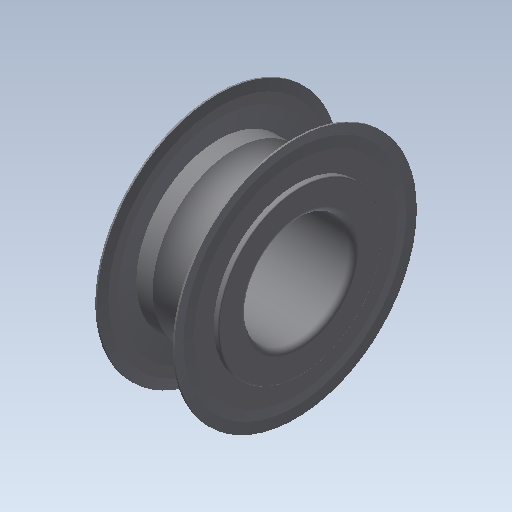
# Autodesk Inventor part: 6201-2Z_PART1
Saved by Autodesk Inventor 2020 (Build 240168000, 168)
## iProperties
Created: 2019-03-20
Part Number: 6201-2Z_PART1
Material: Generic
Catalog Web Link: www.cadenas.de
Description: -Deep groove ball bearings
Vendor: SKF
Document SubType Name: Modeling
Designer: psadmin
Manufacturer: SKF
Mass: 1.48168 g
Surface Area: 25.5062 cm^2
Volume: 1.48168 cm^3
Density: 1 g/cm^3
Appearance: PSOLRGB-175-175-175
Category: PARTsolutions
Company: SKF
PSOL_IDENT_0: {$CADENAS_DATA\23d-libs\skf\bearings_units_and_housings\ball_bearings\deep_groove_ball_bearings\bb1_
PSOL_IDENT_1: 001_101.prj},192 {VTYP=3D},{NB=6201-2Z_PART1},{LINA=6201-2Z_PART1},{NN=BB1_001_101_PART1},{NOPRJ=TRU
PSOL_IDENT_2: E},{DATE=18.03.2019 09:24:30},{GEOMDATE=08.08.2018 12:16:40},{VERSION=},{LINEID=9770},{WBVAR=},{WBNU
PSOL_IDENT_3: MERIC=}  {NB=6201-2Z_PART1},{LINA=6201-2Z_PART1},{KT=DUMMY},{PRODUCTID=1050070201},{DESIGNATION=6201
PSOL_IDENT_4: -2Z},{DD=12.00},{D=32.000},{B=10.000},{C=0.000},{DD1=18.45},{DD2=0.0},{D1=0.00},{D2=27.34},{D3=0.00}
PSOL_IDENT_5: ,{D4=0.000},{HH=MIN},{BB=0.000},{FF=0.00},{R0MAX=MIN},{R0=MIN},{R12=0.60},{PITCH=22.00},{DW=6.000},{
PSOL_IDENT_6: DDAMIN=16.200},{DDAMAX=18.400},{DDBMIN=MIN},{DDBMAX=MIN},{DBMIN=MIN},{DAMAX=27.800},{BBAMIN=MIN},{CA
PSOL_IDENT_7: MAX=MIN},{RAMAX=0.600},{LOAD1=7.280},{LOAD2=3.100},{LOAD3=0.132},{SPEED1=50000},{SPEED2=26000},{KR=0
PSOL_IDENT_8: .025},{F0=12.000},{Z=7},{II=1},{MASS=0.039},{BEARING=6201-2Z},{RING=},{HELP=2.990},{HELP2=2.330},{DD
PSOL_IDENT_9: 1ALG=9.225},{YALG=9.225},{PITCH1=22.000},{DW1=6.000},{YALG1=13.010},{HALG1=2.990},{SH=9.225},{CU=0.8
PSOL_IDENT_10: 00},{DESIGN=dgbbw2z},{HALG=3.225},{B1=0},{ALGO=1.000}
NT: Deep groove ball bearings
NB: 6201-2Z_PART1
NBSYN: $DESIGNATION._PART1
LINA: 6201-2Z_PART1
SUPPLIER: SKF
ARTICLENO: 6201-2Z_PART1
BOMINFO: 6201-2Z_PART1
CREATOR: CADENAS GmbH
Title: 6201-2Z_PART1
Author: Cadenas PARTsolutions
Comments: Deep groove ball bearings
Autodesk Inventor part; units mm, degrees
ref_plane "YZ Plane" through (0, 0, 0) normal (1, 0, 0) x (0, 1, 0)
ref_plane "XZ Plane" through (0, 0, 0) normal (0, 1, 0) x (-1, 0, 0)
ref_plane "XY Plane" through (0, 0, 0) normal (0, 0, 1) x (1, 0, 0)
sketch "Sketch_17" plane through (0, 0, 0) normal (0, 0, 1) x (1, 0, 0)
  line L0 (50, 0) -> (-50, 0)
  line L1 (0, 9.105) -> (0, 6.6)
  arc A0 (0, 6.6) -> (0.6, 6) centre (0.6, 6.6) ccw
  line L2 (0.6, 6) -> (9.4, 6)
  arc A1 (9.4, 6) -> (10, 6.6) centre (9.4, 6.6) ccw
  line L3 (10, 6.6) -> (10, 9.105)
  arc A2 (10, 9.105) -> (9.88, 9.225) centre (9.88, 9.105) ccw
  line L4 (9.88, 9.225) -> (7.4185, 9.225)
  arc A3 (2.5815, 9.225) -> (7.4185, 9.225) centre (5, 11) ccw
  line L5 (2.5815, 9.225) -> (0.12, 9.225)
  arc A4 (0.12, 9.225) -> (0, 9.105) centre (0.12, 9.105) ccw
  constraints: 12 end point, 10 point on circle, 5 centre point
revolve "Revolution1" add sketch "Sketch_17" angle 360 about axis through (50, 0, 0) along (1, 0, 0)
sketch "Sketch_20" plane through (0, 0, 0) normal (0, 0, 1) x (1, 0, 0)
  line L0 (50, 0) -> (-50, 0)
  line L1 (0.54, 13.67) -> (0.63, 12.5563)
  line L2 (0.63, 12.5563) -> (0.54, 11.4425)
  line L3 (0.54, 11.4425) -> (0.54, 9.215)
  line L4 (0.54, 9.215) -> (0.72, 9.215)
  line L5 (0.72, 9.215) -> (0.9, 11.4425)
  line L6 (0.9, 11.4425) -> (0.9, 12.5563)
  line L7 (0.9, 12.5563) -> (0.72, 13.67)
  line L8 (0.72, 13.67) -> (0.54, 13.67)
  constraints: 18 end point
revolve "Revolution2" add sketch "Sketch_20" angle 360 about axis through (50, 0, 0) along (1, 0, 0)
sketch "Sketch_21" plane through (0, 0, 0) normal (0, 0, 1) x (1, 0, 0)
  line L0 (50, 0) -> (-50, 0)
  line L1 (9.1, 12.5563) -> (9.1, 11.4425)
  line L2 (9.1, 11.4425) -> (9.28, 9.215)
  line L3 (9.28, 9.215) -> (9.46, 9.215)
  line L4 (9.46, 9.215) -> (9.46, 11.4425)
  line L5 (9.46, 11.4425) -> (9.37, 12.5563)
  line L6 (9.37, 12.5563) -> (9.46, 13.67)
  line L7 (9.46, 13.67) -> (9.28, 13.67)
  line L8 (9.28, 13.67) -> (9.1, 12.5563)
  constraints: 18 end point
revolve "Revolution3" add sketch "Sketch_21" angle 360 about axis through (50, 0, 0) along (1, 0, 0)
body "Solid1"
